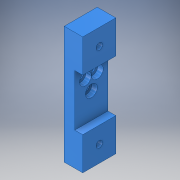
# Autodesk Inventor part: Back_Bracket_40mm
Saved by Autodesk Inventor 2019.4 (Build 234330000, 330)
## iProperties
Created: 2021-02-01
Part Number: Back_Bracket_40mm
Material: ABS Plastic
Document SubType Name: Modeling
Designer: Jorian Brusind
Density: 1.06 g/cm^3
Appearance: Cyan
Mass: 29.0633 g
Surface Area: 97.0192 cm^2
Volume: 27.4182 cm^3
Author: Jorian Brusind
Autodesk Inventor part; units mm, degrees
ref_plane "YZ Plane" through (0, 0, 0) normal (1, 0, 0) x (0, 1, 0)
ref_plane "XZ Plane" through (0, 0, 0) normal (0, 1, 0) x (-1, 0, 0)
ref_plane "XY Plane" through (0, 0, 0) normal (0, 0, 1) x (1, 0, 0)
sketch "Sketch1" plane through (0, 0, 0) normal (0, 1, 0) x (-1, 0, 0)
  line L0 (0, 0) -> (8, 0)
  line L1 (8, 0) -> (8, -25)
  line L2 (8, -25) -> (0, -25)
  line L3 (0, -25) -> (0, 0)
  dimension "d0" = 8
  dimension "d1" = 25
  constraints: 8 end point, 2 parallel, 1 horizontal, 1 perpendicular
  measures "d0" distance of L1.end L2.end
  measures "d1" distance of L0.end L1.end
extrude "Extrusion1" add sketch "Sketch1" along normal blind 89
sketch "Sketch2" plane through (0, 0, 0) normal (1, 0, 0) x (0, 0, -1)
  line L0 (0, 89) -> (25, 89) projected
  line L1 (0, 89) -> (25, 89)
  line L2 (25, 89) -> (25, 64)
  line L3 (25, 64) -> (0, 64)
  line L4 (0, 64) -> (0, 89)
  line L5 (25, 0) -> (25, 89) projected
  line L6 (25, 0) -> (0, 0)
  line L7 (0, 0) -> (0, 25)
  line L8 (0, 25) -> (25, 25)
  line L9 (25, 25) -> (25, 0)
  dimension "d4" = 25
  dimension "d5" = 25
  dimension "d6" = 25
  dimension "d7" = 25
  constraints: 16 end point, 4 parallel, 2 horizontal, 2 perpendicular
  measures "d4" distance of L2.end L3.end
  measures "d5" distance of L1.end L2.end
  measures "d6" distance of L7.end L8.end
  measures "d7" distance of L6.end L7.end
extrude "Extrusion2" add sketch "Sketch2" along normal blind 6
sketch "Sketch3" plane through (6, 0, 0) normal (1, 0, 0) x (0, 0, -1)
  line L0 (0, 0) -> (25, 0) projected
  line L1 (0, 0) -> (12.5, 0)
  line L2 (12.5, 0) -> (12.5, 12.5)
  circle A0 centre (12.5, 12.5) radius 2.5
  circle A1 centre (12.5, 76.5) radius 2.5
  line L3 (25, 89) -> (0, 89) projected
  line L4 (0, 89) -> (0, 64) projected
  dimension "d10" = 12.5
  dimension "d11" = 5
  dimension "d12" = 5
  dimension "d13" = 12.5
  dimension "d14" = 12.5
  constraints: 4 end point, 2 centre point, 1 coincident, 1 midpoint, 1 perpendicular
  measures "d10" distance of L1.end L2.end
  measures "d11" diameter of A0
  measures "d12" diameter of A1
  measures "d13" distance from line of L3 A1.centre
  measures "d14" distance from line of L4 A1.centre
sketch "Sketch4" plane through (0, 25, -25) normal (1, 0, 0) x (0, 0, -1)
  circle A0 centre (-17, 29.5) radius 2.5
  line L0 (-25, -25) -> (0, -25) projected
  line L1 (-25, 0) -> (-25, 39) projected
  circle A1 centre (-8, 29.5) radius 2.5
  line L2 (0, 0) -> (0, 39) projected
  circle A2 centre (-12.5, 19.5) radius 2.5
  circle A3 centre (-12.5, 39.5) radius 2.5
  dimension "d15" = 5
  dimension "d16" = 54.5
  dimension "d17" = 8
  dimension "d18" = 5
  dimension "d19" = 8
  dimension "d20" = 54.5
  dimension "d21" = 5
  dimension "d22" = 5
  dimension "d23" = 10
  dimension "d24" = 4.5
  dimension "d25" = 10
  dimension "d26" = 4.5
  constraints: 4 centre point
  measures "d15" diameter of A0
  measures "d16" distance from line of L0 A0.centre
  measures "d17" distance from line of L1 A0.centre
  measures "d18" diameter of A1
  measures "d19" distance from line of L2 A1.centre
  measures "d20" distance from line of L0 A1.centre
  measures "d21" diameter of A2
  measures "d22" diameter of A3
  measures "d23" vertical distance of A0.centre A3.centre
  measures "d24" horizontal distance of A2.centre A1.centre
  measures "d25" vertical distance of A0.centre A2.centre
  measures "d26" horizontal distance of A1.centre A3.centre
extrude "Extrusion3" cut sketch "Sketch3" against normal up to next
extrude "Extrusion4" cut sketch "Sketch4" against normal up to next
sketch "Sketch5" plane through (0, 25, -25) normal (1, 0, 0) x (0, 0, -1)
  circle A0 centre (-12.5, 39.5) radius 2.5 projected
  circle A1 centre (-12.5, 39.5) radius 4.5
  circle A2 centre (-17, 29.5) radius 2.5 projected
  circle A3 centre (-17, 29.5) radius 4.5
  circle A4 centre (-8, 29.5) radius 2.5 projected
  circle A5 centre (-8, 29.5) radius 4.5
  circle A6 centre (-12.5, 19.5) radius 2.5 projected
  circle A7 centre (-12.5, 19.5) radius 4.5
  point P0 (-25, -25)
  dimension "d31" = 9
  dimension "d32" = 9
  dimension "d33" = 9
  dimension "d34" = 9
  constraints: 4 centre point, 4 coincident
  measures "d31" diameter of A1
  measures "d32" diameter of A3
  measures "d33" diameter of A5
  measures "d34" diameter of A7
extrude "Extrusion5" cut sketch "Sketch5" against normal blind 4
body "Solid1"
